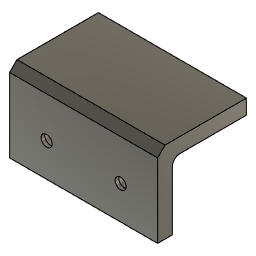
stress_Anal v4 (Autodesk Fusion 360 design; units mm, degrees)
Autodesk Fusion 360 part; units mm, degrees
sketch "Sketch1" plane through (0, 0, 0) normal (1, 0, 0) x (0, 1, 0)
  line L0 (0, 0) -> (10, 0)
  line L1 (10, 0) -> (10, 45)
  line L2 (10, 55) -> (0, 55)
  line L3 (0, 55) -> (0, 0)
  line L4 (0, 55) -> (60, 55)
  line L5 (60, 55) -> (60, 45)
  line L6 (60, 45) -> (10, 45)
  line L7 (0, 45) -> (0, 55)
  constraint horizontal L0
  constraint vertical L1
  constraint horizontal L2
  constraint vertical L3
  constraint coincident L0.start L3.end
  constraint horizontal L4
  constraint vertical L5
  constraint horizontal L6
  constraint vertical L7
extrude "Extrude1" add sketch "Sketch1" along normal mid plane 100
sketch "Sketch2" plane through (0, 10, 0) normal (0, 1, 0) x (-1, 0, 0)
  line L0 (50, 45) -> (-50, 45)
  line L1 (-50, 45) -> (-50, 0)
  line L2 (-50, 0) -> (50, 0)
  line L3 (50, 0) -> (50, 45)
  circle A0 centre (25, 22.5) radius 3.75
  line L4 (0, 0) -> (0, 67.2521)
  circle A1 centre (-25, 22.5) radius 3.75
  dimension "d3" = 7.5
  dimension "d4" = 25
  constraint coincident L4.start origin
  constraint perpendicular L0 L4
  constraint symmetric A0 L4 A1
  measures "d3" diameter of A0
  measures "d4" distance of A0.centre L4
extrude "Extrude2" cut sketch "Sketch2" against normal blind 28 contours A0 | A1
sketch "Sketch3" plane through (0, 10, 0) normal (0, 1, 0) x (-1, 0, 0)
  circle A0 centre (-25, 22.5) radius 3.75
  circle A1 centre (25, 22.5) radius 3.75
  line L0 (50, 45) -> (-50, 45)
  line L1 (-50, 45) -> (-50, 0)
  line L2 (-50, 0) -> (50, 0)
  line L3 (50, 0) -> (50, 45)
  circle A2 centre (-25, 22.5) radius 5
  circle A3 centre (25, 22.5) radius 5
  dimension "d7" = 10
  dimension "d8" = 10
  constraint concentric A0 A2
  constraint concentric A1 A3
  measures "d7" diameter of A2
  measures "d8" diameter of A3
extrude "Extrude3" cut sketch "Sketch3" against normal blind 7.5 contours A2 | A3
fillet "Fillet1" radius 5 1 edges at (0, 10, 45)
chamfer "Chamfer1" distance 5 angle 45 1 edges at (0, 0, 55)
